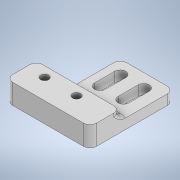
# Autodesk Inventor part: Enstopsupportshoulder
Saved by Autodesk Inventor 2022 (Build 260153000, 153)
## iProperties
Created: 2022-03-17
Part Number: Enstopsupportshoulder
Material: Genérico
Document SubType Name: Modeling
Designer: JK
Density: 1 g/cm^3
Appearance: Valor por defecto
Author: JK
Autodesk Inventor part; units mm, degrees
ref_plane "YZ Plane" through (0, 0, 0) normal (1, 0, 0) x (0, 1, 0)
ref_plane "XZ Plane" through (0, 0, 0) normal (0, 1, 0) x (-1, 0, 0)
ref_plane "XY Plane" through (0, 0, 0) normal (0, 0, 1) x (1, 0, 0)
sketch "Boceto1" plane through (0, 0, 0) normal (0, 1, 0) x (-1, 0, 0)
  line L0 (-8, 12.5) -> (8, 12.5)
  line L1 (8, 12.5) -> (8, -12.5)
  line L2 (8, -12.5) -> (-8, -12.5)
  line L3 (-8, -12.5) -> (-8, 12.5)
  line L4 (-8, 12.5) -> (8, -12.5) construction
  line L5 (8, 12.5) -> (-8, -12.5) construction
  circle A0 centre (-3, -8.5) radius 1.65
  circle A1 centre (4, -8.5) radius 1.65
  line L6 (2.35, -8.5) -> (5.65, -8.5)
  line L7 (5.65, -8.5) -> (5.65, -2.5)
  line L8 (5.65, -2.5) -> (2.35, -2.5)
  line L9 (2.35, -2.5) -> (2.35, -8.5)
  line L10 (-1.35, -8.5) -> (-4.65, -8.5)
  line L11 (-4.65, -8.5) -> (-4.65, -2.5)
  line L12 (-4.65, -2.5) -> (-1.35, -2.5)
  line L13 (-1.35, -2.5) -> (-1.35, -8.5)
  circle A2 centre (4, -2.5) radius 1.65
  circle A3 centre (-3, -2.5) radius 1.65
  point P0 (0, 0)
  point P1 (-4.65, -8.5)
  point P2 (-4.65, -2.5)
  point P3 (5.65, -8.5)
  point P4 (2.35, -2.5)
  dimension "d0" = 3.3
  dimension "d1" = 16
  dimension "d2" = 7
  dimension "d3" = 25
  dimension "d5" = 5
  dimension "d6" = 4
  dimension "d7" = 6
  constraints: 28 end point, 6 parallel, 4 midpoint, 3 horizontal, 3 perpendicular, 2 horizontal alignment, 2 vertical, 12 other
  measures "d1" distance between parallel lines of L1 L3
  measures "d2" distance of point (4, -8.5) point (-3, -8.5)
  measures "d3" distance of L0.end L1.end
  measures "d5" distance from line of point (-3, -8.5) L3
  measures "d6" distance from line of L2 point (4, -8.5)
  measures "d7" distance of L6.end L7.end
extrude "Extrusión1" add sketch "Boceto1" along normal blind 3
sketch "Boceto2" plane through (0, 3, 0) normal (0, 1, 0) x (1, 0, 0)
  line L0 (8, -12.5) -> (8, 12.5) projected
  line L1 (8, -12.5) -> (-17, -12.5)
  line L2 (-17, -12.5) -> (-17, -3.5)
  line L3 (-17, -3.5) -> (8, -3.5)
  line L4 (8, -3.5) -> (8, -12.5)
  point P0 (0, 0)
  point P1 (8, -3.5)
  dimension "d10" = 9
  dimension "d11" = 25
  constraints: 8 end point, 2 parallel, 1 horizontal, 1 perpendicular
  measures "d10" distance of L1.end L2.end
  measures "d11" distance of L2.end L3.end
extrude "Extrusión2" add sketch "Boceto2" along normal blind 3 and the other way blind 3
sketch "Boceto3" plane through (0, 6, 0) normal (0, 1, 0) x (1, 0, 0)
  circle A0 centre (-11.5, -6.5) radius 1.2
  circle A1 centre (-2, -6.5) radius 1.2
  line L0 (8, -12.5) -> (8, -3.5) projected
  line L1 (8, -3.5) -> (-17, -3.5) projected
  point P0 (0, 0)
  dimension "d16" = 2.4
  dimension "d17" = 9.5
  dimension "d18" = 10
  dimension "d19" = 3
  constraints: 2 centre point, 1 equal radius, 1 horizontal alignment
  measures "d16" diameter of A0
  measures "d17" distance of A1.centre A0.centre
  measures "d18" distance from line of A1.centre L0
  measures "d19" distance from line of L1 A0.centre
extrude "Extrusión3" cut sketch "Boceto3" against normal through all
fillet "Empalme1" radius 2 7 edges at (-17, 3, 3.5) (-17, 3, 12.5) (8, 4.5, 3.5) (0, 3, 3.5) (-8, 1.5, -12.5) (8, 1.5, -12.5) (8, 3, 12.5)
sketch "Boceto4" plane through (0, 0, 0) normal (0, -1, 0) x (1, 0, 0)
  circle A0 centre (-11.5, 6.5) radius 1.2 projected
  circle A1 centre (-11.5, 6.5) radius 2.15
  circle A2 centre (-2, 6.5) radius 1.2 projected
  circle A3 centre (-2, 6.5) radius 2.15
  line L0 (-13.9826, 6.5) -> (-12.7413, 8.65)
  line L1 (-12.7413, 8.65) -> (-10.2587, 8.65)
  line L2 (-10.2587, 8.65) -> (-9.0174, 6.5)
  line L3 (-9.0174, 6.5) -> (-10.2587, 4.35)
  line L4 (-10.2587, 4.35) -> (-12.7413, 4.35)
  line L5 (-12.7413, 4.35) -> (-13.9826, 6.5)
  line L6 (-4.4826, 6.5) -> (-3.2413, 8.65)
  line L7 (-3.2413, 8.65) -> (-0.7587, 8.65)
  line L8 (-0.7587, 8.65) -> (0.4826, 6.5)
  line L9 (0.4826, 6.5) -> (-0.7587, 4.35)
  line L10 (-0.7587, 4.35) -> (-3.2413, 4.35)
  line L11 (-3.2413, 4.35) -> (-4.4826, 6.5)
  point P0 (0, 0)
  dimension "d23" = 4.3
  constraints: 24 end point, 4 coincident, 2 centre point, 2 horizontal alignment, 2 tangent, 1 horizontal, 26 other
  measures "d23" diameter of A1
extrude "Extrusión4" cut sketch "Boceto4" against normal blind 4 contours A0 | A1 | A1 L2 L3 | A1 L1 L2 | L3 L4 A1 | A1 L0 L1 | L4 L5 A1 | A1 L5 L0 | A2 | A3 | A3 L8 L9 | A3 L7 L8 | L9 L10 A3 | A3 L6 L7 | L10 L11 A3 | A3 L11 L6
